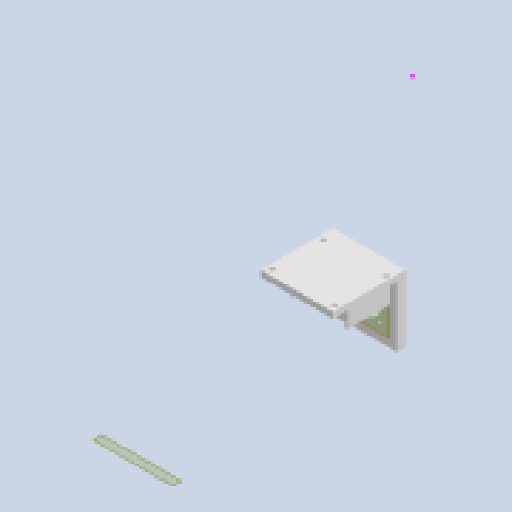
# Autodesk Inventor part: крепление
Saved by Autodesk Inventor 2024.2 (Build 282272000, 272)
## iProperties
Created: 2025-11-21
Part Number: крепление
Material: Типовые
Document SubType Name: Modeling
Designer: katya_notebook
Density: 1 g/cm^3
Appearance: По умолчанию
Author: katya_notebook
Autodesk Inventor part; units mm, degrees
ref_plane "YZ Plane" through (0, 0, 0) normal (1, 0, 0) x (0, 1, 0)
ref_plane "XZ Plane" through (0, 0, 0) normal (0, 1, 0) x (-1, 0, 0)
ref_plane "XY Plane" through (0, 0, 0) normal (0, 0, 1) x (1, 0, 0)
ref_plane "РабПлоскость3" through (-41.0529, -164.837, 166.5004) normal (0, 0, -1) x (-1, 0, 0)
sketch "Эскиз3" plane through (-41.0529, -164.837, 166.5004) normal (0, 0, -1) x (-1, 0, 0)
  circle A0 centre (-0.1829, -8.498) radius 11 projected
  circle A1 centre (-0.1829, -8.498) radius 11
  point P0 (-41.0529, 164.837)
  constraints: 1 centre point, 1 coincident, 1 concentric
ref_plane "РабПлоскость2" through (-41.0529, -164.837, 166.5004) normal (0, 0, -1) x (-1, 0, 0)
sketch "Эскиз4" plane through (-41.0529, -164.837, 166.5004) normal (0, 0, -1) x (-1, 0, 0)
  point P0 (-41.0529, 164.837)
ref_plane "РабПлоскость5" through (-25.5269, -152.335, 167.4504) normal (0, 0, -1) x (-1, 0, 0)
sketch "Эскиз6" plane through (-25.5269, -152.335, 167.4504) normal (0, 0, -1) x (-1, 0, 0)
  circle A0 centre (15.3431, -21) radius 2.6 projected
  line L0 (-14.6569, 0) -> (45.3431, 0)
  line L1 (45.3431, 0) -> (45.3431, -42)
  line L2 (45.3431, -42) -> (-14.6569, -42)
  line L3 (-14.6569, -42) -> (-14.6569, 0)
  line L4 (-14.6569, 0) -> (45.3431, -42) construction
  line L5 (45.3431, 0) -> (-14.6569, -42) construction
  line L6 (45.3431, -42) -> (-14.6569, -42)
  line L7 (-14.6569, -42) -> (-14.6569, -50.705)
  line L8 (-14.6569, -50.705) -> (45.3431, -50.705)
  line L9 (45.3431, -50.705) -> (45.3431, -42)
  circle A1 centre (15.3432, -20.9999) radius 17.4999 projected
  circle A2 centre (15.3435, -20.9998) radius 17.4996 projected
  circle A3 centre (15.3431, -21) radius 2.5 projected
  circle A4 centre (15.3431, -21) radius 17.5
  point P0 (-25.5269, 152.335)
  point P1 (45.3431, -42)
  point P2 (-14.6569, -42)
  point P3 (24.6233, -6.1633)
  point P4 (30.6276, -12.4774)
  point P5 (45.3431, -42)
  point P6 (-14.6569, -42)
  dimension "d9" = 60
  dimension "d10" = 42
  dimension "d11" = 60
  constraints: 20 end point, 4 parallel, 2 horizontal, 2 midpoint, 2 perpendicular, 1 centre point, 1 coincident, 1 collinear
  measures "d9" distance of L1.end L2.end
  measures "d10" distance of L2.end L0.start
  measures "d11" distance of L7.end L8.end
extrude "Выдавливание3" add sketch "Эскиз6" along normal blind 6.5 contours L0 L1 L2 L3 | L2 L9 L8 L7
ref_plane "РабПлоскость6" through (-53.87, -152.335, 177.9504) normal (0, 1, 0) x (1, 0, 0)
sketch "Эскиз7" plane through (-53.87, -152.335, 177.9504) normal (0, 1, 0) x (1, 0, 0)
  line L0 (-17, 17) -> (43, 17) projected
  line L1 (43, 17) -> (-17, 17)
  line L2 (-17, 17) -> (-17, -43)
  line L3 (-17, -43) -> (43, -43)
  line L4 (43, -43) -> (43, 17)
  point P0 (53.87, 177.9504)
  dimension "d16" = 60
  dimension "d17" = 60
  constraints: 8 end point, 2 parallel, 1 horizontal, 1 perpendicular
  measures "d16" distance of L2.end L3.end
  measures "d17" distance of L1.end L2.end
extrude "Выдавливание5" add sketch "Эскиз7" along normal blind 5
sketch "Эскиз8" plane through (-53.87, -152.335, 177.9504) normal (0, -1, 0) x (1, 0, 0)
  line L0 (-17, -10.5) -> (43, -10.5) projected
  line L1 (43, 43) -> (43, -10.5) projected
  line L2 (-17, 43) -> (43, 43) projected
  line L3 (-17, -10.5) -> (-17, 43) projected
  line L4 (-10.5, -10.5) -> (-8.5, -10.5)
  line L5 (-8.5, -10.5) -> (-8.5, 24.5)
  line L6 (-8.5, 24.5) -> (-10.5, 24.5)
  line L7 (-10.5, 24.5) -> (-10.5, -10.5)
  line L8 (34.5, -10.5) -> (36.5, -10.5)
  line L9 (36.5, -10.5) -> (36.5, 24.5)
  line L10 (36.5, 24.5) -> (34.5, 24.5)
  line L11 (34.5, 24.5) -> (34.5, -10.5)
  point P0 (53.87, -177.9504)
  point P1 (-8.5, -10.5)
  point P2 (36.5, -10.5)
  dimension "d20" = 2
  dimension "d21" = 6.5
  dimension "d22" = 35
  dimension "d23" = 35
  dimension "d24" = 2
  dimension "d25" = 6.5
  constraints: 16 end point, 4 parallel, 2 horizontal, 2 perpendicular, 2 point on line
  measures "d20" distance of L5.end L6.end
  measures "d21" distance between parallel lines of L3 L7
  measures "d22" distance of L6.end L4.start
  measures "d23" distance of L8.end L9.end
  measures "d24" distance of L9.end L10.end
  measures "d25" distance between parallel lines of L1 L9
extrude "Выдавливание6" add sketch "Эскиз8" along normal blind 20 contours L7 L6 L5 L0 | L11 L10 L9 L0
sketch "Эскиз9" plane through (-53.87, -152.335, 177.9504) normal (0, -1, 0) x (1, 0, 0)
  circle A0 centre (-13, 38) radius 2
  circle A1 centre (39, 38) radius 2
  circle A2 centre (-13, -4.5) radius 2
  circle A3 centre (39, -4.5) radius 2
  line L0 (-17, 43) -> (43, 43) projected
  line L1 (-17, -10.5) -> (-17, 43) projected
  line L2 (43, 43) -> (43, -10.5) projected
  line L3 (43, -10.5) -> (-17, -10.5) projected
  point P0 (53.87, -177.9504)
  dimension "d28" = 4
  dimension "d29" = 4
  dimension "d30" = 4
  dimension "d31" = 4
  dimension "d32" = 5
  dimension "d33" = 4
  dimension "d34" = 5
  dimension "d35" = 4
  dimension "d36" = 4
  dimension "d37" = 4
  dimension "d38" = 6
  dimension "d39" = 6
  constraints: 4 centre point
  measures "d28" diameter of A0
  measures "d29" diameter of A1
  measures "d30" diameter of A2
  measures "d31" diameter of A3
  measures "d32" distance from line of L0 A0.centre
  measures "d33" distance from line of L1 A0.centre
  measures "d34" distance from line of L0 A1.centre
  measures "d35" distance from line of L2 A1.centre
  measures "d36" distance from line of L2 A3.centre
  measures "d37" distance from line of L1 A2.centre
  measures "d38" distance from line of A3.centre L3
  measures "d39" distance from line of A2.centre L3
extrude "Выдавливание7" cut sketch "Эскиз9" against normal blind 20 contours A0 | A1 | A2 | A3
sketch "Эскиз10" plane through (-25.5269, -152.335, 160.9504) normal (0, 0, -1) x (-1, 0, 0)
  circle A0 centre (-0.1569, -36.5) radius 1.2645 projected
  circle A1 centre (30.8431, -36.5) radius 1.2645 projected
  circle A2 centre (-0.1569, -5.5) radius 1.2645 projected
  circle A3 centre (30.8431, -5.5) radius 1.2645 projected
  circle A4 centre (-0.1569, -36.5) radius 1.2645
  circle A5 centre (-0.1569, -5.5) radius 1.2645
  circle A6 centre (30.8431, -5.5) radius 1.2645
  circle A7 centre (30.8431, -36.5) radius 1.2645
  point P0 (-25.5269, 152.335)
  constraints: 4 centre point, 4 coincident, 4 concentric
extrude "Выдавливание8" cut sketch "Эскиз10" against normal blind 20
ref_plane "РабПлоскость7" through (-10.87, -203.04, 349.4504) normal (0, -1, 0) x (1, 0, 0)
sketch "Эскиз11" plane through (-10.87, -203.04, 349.4504) normal (0, -1, 0) x (1, 0, 0)
  circle A0 centre (-12, -185.25) radius 1.75 projected
  circle A1 centre (-30, -185.25) radius 1.75 projected
  circle A2 centre (-48, -185.25) radius 1.75 projected
  circle A3 centre (-12, -185.25) radius 1.75
  circle A4 centre (-30, -185.25) radius 1.75
  circle A5 centre (-48, -185.25) radius 1.75
  point P0 (10.87, -349.4504)
  constraints: 3 centre point, 3 coincident, 3 concentric
extrude "Выдавливание9" cut sketch "Эскиз11" against normal blind 10
